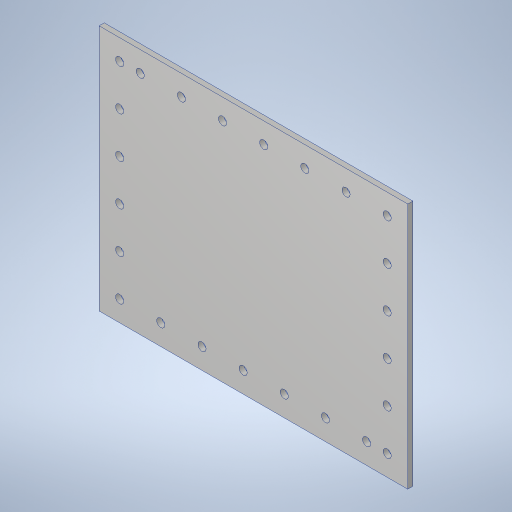
# Autodesk Inventor part: EL2-C-003
Saved by Autodesk Inventor 2023.4 (Build 274418000, 418)
## iProperties
RuleStatus: InUse
Created: 2025-01-11
Part Number: EL2-C-003
Material: Aluminum 6061
Document SubType Name: Modeling
Designer: brand
Mass: 132.735 g
Surface Area: 177.419 cm^2
Volume: 49.1612 cm^3
Density: 2.7 g/cm^3
Appearance: Aluminum - Flat
AfterDocNew0: SHOW
AfterDocOpen0: SHOW
Author: brand
Autodesk Inventor part; units mm, degrees
ref_plane "YZ Plane" through (0, 0, 0) normal (1, 0, 0) x (0, 1, 0)
ref_plane "XZ Plane" through (0, 0, 0) normal (0, 1, 0) x (-1, 0, 0)
ref_plane "XY Plane" through (0, 0, 0) normal (0, 0, 1) x (1, 0, 0)
sketch "Sketch1" plane through (0, 0, 0) normal (0, 0, 1) x (1, 0, 0)
  line L0 (-95.25, -76.2) -> (95.25, -76.2)
  line L1 (95.25, -76.2) -> (95.25, 76.2)
  line L2 (95.25, 76.2) -> (-95.25, 76.2)
  line L3 (-95.25, 76.2) -> (-95.25, -76.2)
  line L4 (-95.25, -76.2) -> (95.25, 76.2) construction
  line L5 (95.25, -76.2) -> (-95.25, 76.2) construction
  point P0 (0, 0)
  dimension "width" = 190.5
  dimension "length" = 152.4
  constraints: 12 end point, 2 midpoint, 2 parallel, 1 horizontal, 1 perpendicular
  measures "width" distance of L2.end L1.end
  measures "length" distance of L0.end L1.end
extrude "Extrusion1" add sketch "Sketch1" along normal mid plane 3.175
sketch "Sketch2" plane through (0, 0, 1.5875) normal (0, 0, 1) x (1, 0, 0)
  line L0 (-95.25, -76.2) -> (-95.25, 76.2) construction
  line L1 (-95.25, 76.2) -> (95.25, 76.2) construction
  line L2 (95.25, 76.2) -> (95.25, -76.2) construction
  line L3 (95.25, -76.2) -> (-95.25, -76.2) construction
  point P0 (0, 0)
  point P1 (-82.55, -63.5)
  point P2 (82.55, 63.5)
  dimension "d4" = 12.7
  dimension "d5" = 12.7
  dimension "d19" = 12.7
  dimension "d20" = 12.7
  measures "d4" distance from line of L0 point (-82.55, -63.5)
  measures "d5" distance from line of L3 point (-82.55, -63.5)
  measures "d19" distance from line of L2 point (82.55, 63.5)
  measures "d20" distance from line of L1 point (82.55, 63.5)
hole "Hole1" at (-82.55, -63.5, 1.5875) direction (0, 0, -1) diameter 5.1054 end through all clearance for "Flat Head Machine Screw (82)" size "#10" standard "Ansi Unified Screw Threads"
pattern_linear "Rectangular Pattern1" count 8 spacing 25.4 along (0, 1, 0) of "Hole1"
pattern_linear "Rectangular Pattern2" count 7 spacing 25.4 along (1, 0, 0) of "Hole1"
hole "Hole2" at (82.55, 63.5, 1.5875) direction (0, 0, -1) diameter 5.1054 end through all clearance for "Flat Head Machine Screw (82)" size "#10" standard "Ansi Unified Screw Threads"
pattern_linear "Rectangular Pattern3" count 7 spacing 25.4 along (-1, 0, 0) of "Hole2"
pattern_linear "Rectangular Pattern4" count 7 spacing 25.4 along (0, -1, 0) of "Hole2"
equation "\"d19\" = d4"
equation "\"d20\" = d5"
body "Solid1"
